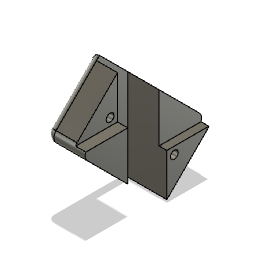
stepper mount v9 (Autodesk Fusion 360 design; units mm, degrees)
Autodesk Fusion 360 part; units mm, degrees
sketch "motor face" plane through (0, 0, 0) normal (0, 1, 0) x (1, 0, 0)
  circle A0 centre (0, 0) radius 14
  line L0 (0, 0) -> (37.537965, 0) construction
  circle A1 centre (17.5, 0) radius 2
  line L1 (17.5, 3.5) -> (13.555442, 3.5)
  line L2 (17.5, -3.5) -> (13.555442, -3.5)
  line L3 (0, 0) -> (0, 22.721675) construction
  circle A2 centre (0, 8) radius 4.5
  circle A3 centre (-17.5, 0) radius 2
  line L4 (-17.5, 3.5) -> (-13.555442, 3.5)
  line L5 (-17.5, -3.5) -> (-13.555442, -3.5)
  arc A4 (17.5, -3.5) -> (17.5, 3.5) centre (17.5, 0) ccw
  arc A5 (-17.5, 3.5) -> (-17.5, -3.5) centre (-17.5, 0) ccw
  line L6 (0, 0) -> (0, -28.412749) construction
  line L7 (0, -18) -> (8.8, -18)
  line L8 (8.8, -18) -> (8.8, -10.888526)
  line L9 (-8.8, -18) -> (-8.8, -10.888526)
  line L10 (0, -18) -> (-8.8, -18)
  circle A6 centre (0, 8) radius 2.46
  line L11 (-0.98, 10.256369) -> (-0.98, 5.743631)
  line L12 (0.98, 10.256369) -> (0.98, 5.743631)
  point P0 (0, 14)
  point P1 (0, 3.5)
  dimension "d1" = 28
  dimension "d2" = 4
  dimension "d3" = 17.5
  dimension "d4" = 7
  dimension "d5" = 9
  dimension "d6" = 10.5
  dimension "d7" = 8.8
  dimension "d8" = 32
  dimension "d11" = 4.92
  dimension "d12" = 0.98
  constraint coincident A0.centre L0.start
  constraint horizontal L0
  constraint coincident L0 A1.centre
  constraint concentric A1 A4
  constraint tangent L1 A4
  constraint horizontal L1
  constraint tangent L2 A4
  constraint parallel L1 L2
  constraint perpendicular L0 L3
  constraint coincident L3 A2.centre
  constraint coincident A0 P0
  constraint coincident L3 P0
  constraint coincident A2 P1
  constraint coincident L3 P1
  constraint symmetric A1 L3 A3
  constraint symmetric L3 A4 A5
  constraint symmetric L1.start L3 L4.start
  constraint symmetric L2.start L3 L5.start
  constraint perpendicular L0 L6
  constraint coincident L6 L7.start
  constraint perpendicular L6 L7
  constraint perpendicular L7 L8
  constraint symmetric L6 L7.start L10.start
  constraint symmetric L6 L7.end L9.start
  constraint concentric A2 A6
  constraint vertical L11
  measures "d1" diameter of A0
  measures "d2" diameter of A1
  measures "d3" distance of A0.centre A1.centre
  measures "d4" diameter of A4
  measures "d5" diameter of A2
  measures "d6" distance of P0 P1
  measures "d7" distance of L7.start L7.end
  measures "d8" distance of P0 L7
  measures "d11" diameter of A6
  measures "d12" distance of L3 L11
extrude "Extrude1" add sketch "motor face" along normal blind 19.3 contours A0 | A0 L7 L8 L9 L10 | A2 | A6 L12 | A6 L11 L12 | A6 L11 picked at (0.744544, -8.119418) picked at (4.18656, -16.495242) picked at (0, 11.811611) picked at (1.181596, 7.372833) picked at (-0.326667, 8.752123) picked at (-1.666309, 8.243546) makes body 1
extrude "Extrude2" add sketch "motor face" along normal blind 0.8 contours A0 L1 L2 A4 | A0 L4 L5 A5 picked at (15.851814, 2.910684) picked at (-15.851814, 2.910684) bodies 1
extrude "Extrude3" add sketch "motor face" against normal blind 1.34 contours A2 | A6 L12 | A6 L11 L12 | A6 L11 picked at (0, 11.811611) picked at (1.181596, 7.372833) picked at (-0.326667, 8.752123) picked at (-1.666309, 8.243546) bodies 1
extrude "Extrude4" add sketch "motor face" against normal blind 3.43 contours A6 L12 | A6 L11 L12 | A6 L11 picked at (1.181596, 7.372833) picked at (-0.326667, 8.752123) picked at (-1.666309, 8.243546) bodies 1
extrude "Extrude5" add sketch "motor face" against normal blind 9.43 contours A6 L11 L12 picked at (-0.326667, 8.752123) bodies 1
sketch "motor clamp face" plane through (0, 0, 0) normal (0, 1, 0) x (1, 0, 0)
  circle A0 centre (17.5, 0) radius 2
  line L0 (17.5, 3.5) -> (13.555442, 3.5)
  arc A1 (17.5, -3.5) -> (17.5, 3.5) centre (17.5, 0) ccw
  line L1 (17.5, -3.5) -> (13.555442, -3.5)
  arc A2 (13.555442, 3.5) -> (-13.555442, 3.5) centre (0, 0) ccw
  arc A3 (-13.555442, -3.5) -> (-8.8, -10.888526) centre (0, 0) ccw
  arc A4 (8.8, -10.888526) -> (13.555442, -3.5) centre (0, 0) ccw
  circle A5 centre (-17.5, 0) radius 2
  line L2 (-17.5, -3.5) -> (-13.555442, -3.5)
  arc A6 (-17.5, 3.5) -> (-17.5, -3.5) centre (-17.5, 0) ccw
  line L3 (-17.5, 3.5) -> (-13.555442, 3.5)
  line L4 (8.8, -18) -> (-8.8, -18)
  line L5 (-8.8, -18) -> (-8.8, -10.888526)
  line L6 (8.8, -18) -> (8.8, -10.888526)
  circle A7 centre (0, 0) radius 22
  line L7 (-22, 10) -> (22, 10)
  line L8 (22, 10) -> (22, -10)
  line L9 (22, -10) -> (-22, -10)
  line L10 (-22, -10) -> (-22, 10)
  line L11 (-22, 10) -> (22, -10) construction
  line L12 (22, 10) -> (-22, -10) construction
  circle A8 centre (17.5, 0) radius 1.25
  circle A9 centre (-17.5, 0) radius 1.25
  dimension "d21" = 20
  dimension "d25" = 44
  dimension "d27" = 2.5
  dimension "d28" = 2.5
  constraint concentric A2 A7
  constraint horizontal L7
  constraint perpendicular L7 L8
  constraint parallel L7 L9
  constraint parallel L8 L10
  constraint coincident L11 A2.centre
  constraint coincident L12 A2.centre
  constraint coincident A2.centre A3.centre
  constraint tangent A7 L10
  constraint concentric A0 A8
  constraint concentric A5 A9
  measures "d21" distance of L7.end L8.end
  measures "d25" distance of L7.start L7.end
  measures "d27" diameter of A8
  measures "d28" diameter of A9
extrude "Extrude6" add sketch "motor clamp face" along normal blind 40 separate body contours A0 | L0 A1 L1 A2 A3 A4 L2 A6 L3 L7 L9 | L0 A1 L1 A2 A4 A7 L7 L9 | A2 A3 L2 A6 L3 A7 L7 L9 | A5 | A8 | A9 picked at (19.2379, -0.161462) picked at (-3.265986, 3.333333) picked at (16.684362, -6.267352) picked at (-16.684362, -6.267352) picked at (-15.7621, -0.161462) picked at (17.867018, -0.068883) picked at (-17.132982, -0.068883) makes body 2
combine "Combine1" operation cut target body 2 tool bodies 1 keep tools
move_face "OffsetFaces1" offset -0.3 9 faces at (12.790197, 12.866667, 5.693053) (-3.265986, 19.3, -3.333333) (16.185147, 0.266667, 3.5) (19.325023, 0.266667, -2.986518) (16.185147, 0.266667, -3.5) (-12.790197, 12.866667, -5.693053) (-16.185147, 0.266667, -3.5) (-19.325023, 0.266667, 2.986518) (-16.185147, 0.266667, 3.5) on bodies 2
move_face "OffsetFaces2" offset -0.8 2 faces at (-16.978792, 0, -0.179043) (18.166667, 0, 0.578512) on bodies 2
extrude "Extrude7" cut sketch "motor clamp face" along normal blind 20 contours A8 | A9 picked at (17.867018, -0.068883) picked at (-17.132982, -0.068883) bodies 2
sketch "bar clamp face" plane through (0, 40, 0) normal (0, 1, 0) x (-1, 0, 0)
  arc A0 (19.595918, -10) -> (19.595918, 10) centre (0, 0) ccw
  line L0 (19.595918, 10) -> (-19.595918, 10)
  arc A1 (-19.595918, 10) -> (-19.595918, -10) centre (0, 0) ccw
  line L1 (-19.595918, -10) -> (19.595918, -10)
  line L2 (-6.35, 6.35) -> (6.35, 6.35)
  line L3 (6.35, 6.35) -> (6.35, -6.35)
  line L4 (6.35, -6.35) -> (-6.35, -6.35)
  line L5 (-6.35, -6.35) -> (-6.35, 6.35)
  line L6 (-6.35, 6.35) -> (6.35, -6.35) construction
  line L7 (6.35, 6.35) -> (-6.35, -6.35) construction
  line L8 (-22, 0.5) -> (22, 0.5)
  line L9 (22, 0.5) -> (22, -0.5)
  line L10 (22, -0.5) -> (-22, -0.5)
  line L11 (-22, -0.5) -> (-22, 0.5)
  line L12 (-22, 0.5) -> (22, -0.5) construction
  line L13 (22, 0.5) -> (-22, -0.5) construction
  dimension "d33" = 12.7
  dimension "d34" = 12.7
  dimension "d35" = 1
  constraint horizontal L2
  constraint perpendicular L2 L3
  constraint parallel L2 L4
  constraint parallel L3 L5
  constraint coincident L6 A0.centre
  constraint coincident L7 A0.centre
  constraint coincident A0.centre A1.centre
  constraint horizontal L8
  constraint perpendicular L8 L9
  constraint parallel L8 L10
  constraint parallel L9 L11
  constraint coincident L12 A0.centre
  constraint coincident L13 A0.centre
  constraint tangent A1 L11
  measures "d33" distance of L3.end L4.end
  measures "d34" distance of L2.end L3.end
  measures "d35" distance of L8.end L9.end
extrude "Extrude8" cut sketch "bar clamp face" against normal up to surface (20.4 mm away) contours A0 L3 L8 L10 | L3 L5 L8 L10 | L3 L4 L5 L10 | A1 L5 L8 L10 | L2 L3 L5 L8 picked at (11.566667, 0) picked at (2.116667, -0.166667) picked at (-2.116667, -2.45) picked at (-11.566667, 0) picked at (2.116667, 2.45) bodies 2
sketch "bar clamp bolts" plane through (0, 0, -10) normal (0, 0, -1) x (-1, 0, 0)
  line L0 (-10.222035, 0) -> (-10.222035, 19.6)
  line L1 (-10.222035, 19.6) -> (10.222035, 19.6)
  line L2 (10.222035, 19.6) -> (10.222035, 0)
  line L3 (10.222035, 0) -> (19.595918, 0)
  line L4 (19.595918, 0) -> (19.595918, 40)
  line L5 (19.595918, 40) -> (-19.595918, 40)
  line L6 (-19.595918, 40) -> (-19.595918, 0)
  line L7 (-19.595918, 0) -> (-10.222035, 0)
  line L8 (-6.35, 19.6) -> (6.35, 19.6)
  line L9 (6.35, 19.6) -> (6.35, 40)
  line L10 (6.35, 40) -> (-6.35, 40)
  line L11 (-6.35, 40) -> (-6.35, 19.6)
  circle A0 centre (-11.493103, 31) radius 1.6
  circle A1 centre (-11.493103, 31) radius 3
  line L12 (-11.493103, 31) -> (-11.493103, 34) construction
  line L13 (-11.493103, 31) -> (-8.35, 31) construction
  line L14 (0, 1.75) -> (0, 22.5)
  circle A2 centre (11.493103, 31) radius 1.6
  circle A3 centre (11.493103, 31) radius 3
  point P0 (-8.493103, 31)
  point P1 (-11.493103, 34)
  dimension "d38" = 3.2
  dimension "d39" = 6
  dimension "d40" = 6
  dimension "d41" = 2
  constraint concentric A0 A1
  constraint vertical L12
  constraint perpendicular L12 L13
  constraint symmetric A0 L14 A2
  constraint symmetric A1 L14 A3
  measures "d38" diameter of A0
  measures "d39" diameter of A1
  measures "d41" distance of L11 L13.end
extrude "Extrude9" cut sketch "bar clamp bolts" against normal up to surface (20 mm away) contours A0 | A2 picked at (-11.453247, 30.608082) picked at (11.532959, 30.608082) bodies 2
extrude "Extrude10" cut sketch "bar clamp bolts" against normal blind 1 contours A1 | A3 picked at (-8.976895, 30.771469) picked at (14.00931, 30.771469) bodies 2
sketch "bar clamp nuts" plane through (0, 0, 10) normal (0, 0, 1) x (1, 0, 0)
  circle A0 centre (11.493103, 31) radius 1.6
  circle A1 centre (-11.493103, 31) radius 1.6
  line L0 (10.222035, 19.6) -> (10.222035, 0)
  line L1 (10.222035, 0) -> (19.595918, 0)
  line L2 (19.595918, 0) -> (19.595918, 40)
  line L3 (19.595918, 40) -> (-19.595918, 40)
  line L4 (-19.595918, 40) -> (-19.595918, 0)
  line L5 (-19.595918, 0) -> (-10.222035, 0)
  line L6 (-10.222035, 0) -> (-10.222035, 19.6)
  line L7 (-10.222035, 19.6) -> (10.222035, 19.6)
  circle A2 centre (-11.493103, 31) radius 3
  circle A3 centre (11.493103, 31) radius 3
  dimension "d46" = 6
  dimension "d47" = 6
  constraint concentric A1 A2
  constraint concentric A0 A3
  measures "d46" diameter of A2
  measures "d47" diameter of A3
extrude "Extrude11" cut sketch "bar clamp nuts" against normal blind 1 contours A2 | A3 picked at (-8.970939, 30.850958) picked at (14.00931, 30.771469) bodies 2
chamfer "Chamfer1" distance 1 angle 45 6 edges at (0, 40, -6.35) (-6.35, 40, -3.425) (6.35, 40, -3.425) (6.35, 40, 3.425) (0, 40, 6.35) (-6.35, 40, 3.425) on bodies 2
fillet "Fillet1" radius 4 10 edges at (19.595918, 20, -10) (-19.595918, 20, -10) (0, 40, -10) (19.595918, 20, 10) (21.330715, 40, 5.385219) (21.330715, 40, -5.385219) (0, 40, 10) (-19.595918, 20, 10) (-21.330715, 40, -5.385219) (-21.330715, 40, 5.385219) on bodies 2
extrude "Extrude12" add sketch "bar clamp face" along normal blind 100 separate body contours L3 L5 L8 L10 | L3 L4 L5 L10 | L2 L3 L5 L8 picked at (2.116667, -0.166667) picked at (-2.116667, -2.45) picked at (2.116667, 2.45) makes body 3
sketch "v bar" plane through (0, 0, 6.35) normal (0, 0, 1) x (1, 0, 0)
  line L0 (-6.35, 40) -> (6.35, 40)
  line L1 (6.35, 40) -> (6.35, 140)
  line L2 (6.35, 140) -> (-6.35, 140)
  line L3 (-6.35, 140) -> (-6.35, 40)
  line L4 (19.05, 90) -> (6.35, 90)
  line L5 (6.35, 90) -> (6.35, 102.7)
  line L6 (6.35, 102.7) -> (19.05, 102.7)
  line L7 (19.05, 102.7) -> (19.05, 90)
  line L8 (19.05, 90) -> (6.35, 102.7) construction
  line L9 (6.35, 90) -> (19.05, 102.7) construction
  line L10 (6.35, 40) -> (-6.35, 40)
  point P0 (12.7, 96.35)
  dimension "d55" = 12.7
  dimension "d56" = 12.7
  dimension "d57" = 50
  constraint horizontal L4
  constraint perpendicular L4 L5
  constraint parallel L4 L6
  constraint parallel L5 L7
  constraint coincident L8 P0
  constraint coincident L9 P0
  constraint collinear L1 L5
  measures "d55" distance of L5.end L6.end
  measures "d56" distance of L4.end L5.end
  measures "d57" distance of L4 L10
extrude "Extrude13" add sketch "v bar" along normal mid plane 100 separate body contours L1 L4 L5 L6 L7 picked at (10.583333, 98.466667) makes body 4
sketch "A clamp bolts" plane through (6.35, 0, 0) normal (1, 0, 0) x (0, 0, -1)
  line L0 (-6.35, 40) -> (6.35, 40)
  line L1 (6.35, 40) -> (6.35, 140)
  line L2 (6.35, 140) -> (-6.35, 140)
  line L3 (-6.35, 140) -> (-6.35, 40)
  line L4 (43.65, 102.7) -> (-56.35, 102.7)
  line L5 (-56.35, 102.7) -> (-56.35, 90)
  line L6 (-56.35, 90) -> (43.65, 90)
  line L7 (43.65, 90) -> (43.65, 102.7)
  circle A0 centre (11.35, 107.7) radius 3 construction
  circle A1 centre (11.35, 107.7) radius 1.6
  line L8 (6.35, 112.7) -> (16.35, 112.7)
  line L9 (16.35, 112.7) -> (16.35, 102.7)
  line L10 (0, 40) -> (0, 140) construction
  line L11 (-56.35, 96.35) -> (43.65, 96.35) construction
  line L12 (-6.35, 112.7) -> (-16.35, 112.7)
  line L13 (-16.35, 112.7) -> (-16.35, 102.7)
  circle A2 centre (-11.35, 107.7) radius 1.6
  circle A3 centre (-11.35, 85) radius 1.6
  line L14 (-6.35, 80) -> (-16.35, 80)
  line L15 (-16.35, 80) -> (-16.35, 90)
  line L16 (6.35, 80) -> (16.35, 80)
  circle A4 centre (11.35, 85) radius 1.6
  line L17 (16.35, 80) -> (16.35, 90)
  line L18 (6.35, 112.7) -> (-6.35, 112.7)
  line L19 (16.35, 102.7) -> (16.35, 90)
  line L20 (6.35, 80) -> (-6.35, 80)
  line L21 (-16.35, 102.7) -> (-16.35, 90)
  circle A5 centre (-11.35, 107.7) radius 3
  circle A6 centre (11.35, 85) radius 3
  line L22 (-14.1, 83.412287) -> (-11.35, 81.824574)
  line L23 (-11.35, 81.824574) -> (-8.6, 83.412287)
  line L24 (-8.6, 83.412287) -> (-8.6, 86.587713)
  line L25 (-8.6, 86.587713) -> (-11.35, 88.175426)
  line L26 (-11.35, 88.175426) -> (-14.1, 86.587713)
  line L27 (-14.1, 86.587713) -> (-14.1, 83.412287)
  line L28 (8.6, 106.112287) -> (11.35, 104.524574)
  line L29 (11.35, 104.524574) -> (14.1, 106.112287)
  line L30 (14.1, 106.112287) -> (14.1, 109.287713)
  line L31 (14.1, 109.287713) -> (11.35, 110.875426)
  line L32 (11.35, 110.875426) -> (8.6, 109.287713)
  line L33 (8.6, 109.287713) -> (8.6, 106.112287)
  point P0 (8.35, 107.7)
  point P1 (11.35, 104.7)
  point P2 (11.35, 110.7)
  point P3 (14.35, 107.7)
  point P4 (-11.35, 85)
  point P5 (11.35, 107.7)
  dimension "d60" = 6
  dimension "d61" = 3.2
  dimension "d62" = 2
  dimension "d63" = 2
  dimension "d64" = 2
  dimension "d65" = 2
  dimension "d71" = 6
  dimension "d72" = 6
  dimension "d73" = 2.75
  dimension "d74" = 2.75
  constraint concentric A0 A1
  constraint coincident A0 P0
  constraint coincident A0 P1
  constraint coincident L1 L8.start
  constraint perpendicular L1 L8
  constraint coincident L4 L9.end
  constraint perpendicular L4 L9
  constraint coincident A0 P2
  constraint coincident A0 P3
  constraint midpoint L0 L10.start
  constraint midpoint L2 L10.end
  constraint midpoint L5 L11.start
  constraint midpoint L7 L11.end
  constraint symmetric A1 L10 A2
  constraint symmetric L8.start L10 L12.start
  constraint symmetric L8.end L10 L12.end
  constraint symmetric L9.end L10 L13.end
  constraint symmetric A1 L11 A4
  constraint symmetric L8.start L11 L16.start
  constraint symmetric L8.end L11 L16.end
  constraint symmetric L9.end L11 L17.end
  constraint symmetric L11 L12.start L14.start
  constraint symmetric L11 L12.end L14.end
  constraint symmetric L11 L13.end L15.end
  constraint symmetric L11 A2 A3
  constraint concentric A2 A5
  constraint concentric A4 A6
  constraint coincident P4 A3.centre
  constraint coincident P5 A0.centre
  measures "d60" diameter of A0
  measures "d61" diameter of A1
  measures "d62" distance of L1 P0
  measures "d63" distance of L4 P1
  measures "d64" distance of L9 P3
  measures "d65" distance of L8 P2
  measures "d71" diameter of A5
  measures "d72" diameter of A6
  measures "d73" distance of P4 L27
  measures "d74" distance of P5 L33
extrude "Extrude14" add sketch "A clamp bolts" along normal blind 15.7 separate body contours L3 L6 L14 L15 | L1 L3 L6 L20 | L1 L6 L16 L17 | L3 L4 L6 L21 | L1 L3 L4 L6 | L1 L4 L6 L19 | L3 L4 L12 L13 | L1 L3 L4 L18 | L1 L4 L8 L9 | A5 | A6 | L22 L23 L24 L25 L26 L27 | L28 L29 L30 L31 L32 L33 picked at (-15.6, 84.470762) picked at (2.116667, 83.333333) picked at (11.27527, 80.669463) picked at (-13.016667, 94.233333) picked at (-2.116667, 98.466667) picked at (13.016667, 98.466667) picked at (-11.42473, 103.369463) picked at (-2.116667, 109.366667) picked at (7.1, 107.170762) picked at (-9.012942, 106.739956) picked at (13.687058, 84.039956) picked at (-10.166667, 82.950407) picked at (12.533333, 109.749593) makes body 5
combine "Combine2" operation cut target body 5 tool bodies 4 keep tools
move_face "OffsetFaces3" offset -0.3 2 faces at (6.35, 81.170201, 3.588485) (6.35, 103.870201, 3.588485) on bodies 5
fillet "Fillet2" radius 3 8 edges at (14.35, 112.7, 16.35) (22.05, 96.35, 16.35) (22.05, 112.7, 0) (22.05, 80, 0) (14.35, 80, 16.35) (14.35, 80, -16.35) (22.05, 96.35, -16.35) (14.35, 112.7, -16.35) on bodies 5
extrude "Extrude15" cut sketch "A clamp bolts" along normal blind 20 from surface at 11 contours A5 | A6 | L22 L23 L24 L25 L26 L27 | L28 L29 L30 L31 L32 L33 picked at (-9.012942, 106.739956) picked at (13.687058, 84.039956) picked at (-10.166667, 82.950407) picked at (12.533333, 109.749593) bodies 5
mirror "Mirror1" about plane through (6.35, 90, 6.35) normal (-1, 0, 0) of bodies 5 makes body 6
sketch "B clamp" plane through (6.35, 0, 0) normal (-1, 0, 0) x (0, 0, 1)
  line L0 (-43.65, 90) -> (56.35, 90)
  line L1 (56.35, 90) -> (56.35, 102.7)
  line L2 (56.35, 102.7) -> (-43.65, 102.7)
  line L3 (-43.65, 102.7) -> (-43.65, 90)
  line L4 (-43.65, 102.7) -> (-43.65, 90)
  line L5 (56.35, 102.7) -> (-43.65, 102.7)
  line L6 (56.35, 90) -> (56.35, 102.7)
  line L7 (-43.65, 90) -> (56.35, 90)
  line L8 (-6.35, 40) -> (6.35, 40)
  line L9 (-6.35, 40) -> (-6.35, 140)
  line L10 (6.35, 140) -> (-6.35, 140)
  line L11 (6.35, 40) -> (6.35, 140)
  circle A0 centre (9.35, 105.7) radius 3
  line L12 (-43.65, 96.35) -> (56.35, 96.35) construction
  line L13 (0, 140) -> (0, 40) construction
  line L14 (0, 96.35) -> (49.007667, 47.342333) construction
  line L15 (9.885534, 86.464466) -> (35.405807, 111.984739)
  line L16 (0, 96.35) -> (34.507271, 130.857271) construction
  line L17 (15.006854, 111.356854) -> (24.892388, 101.47132)
  circle A1 centre (9.35, 105.7) radius 1.6
  circle A2 centre (9.35, 105.7) radius 1.1
  line L18 (-9.885534, 106.235534) -> (15.634739, 131.755807)
  line L19 (15.006854, 111.356854) -> (5.12132, 121.242388)
  line L20 (9.885534, 86.464466) -> (-15.634739, 60.944193)
  line L21 (-15.006854, 81.343146) -> (-5.12132, 71.457612)
  line L22 (-9.885534, 106.235534) -> (-35.405807, 80.715261)
  circle A3 centre (-9.35, 87) radius 3
  circle A4 centre (-9.35, 87) radius 1.6
  circle A5 centre (-9.35, 87) radius 1.1
  line L23 (-15.006854, 81.343146) -> (-24.892388, 91.22868)
  line L24 (6.35, 103.967949) -> (9.35, 102.235898)
  line L25 (9.35, 102.235898) -> (12.35, 103.967949)
  line L26 (12.35, 103.967949) -> (12.35, 107.432051)
  line L27 (12.35, 107.432051) -> (9.35, 109.164102)
  line L28 (9.35, 109.164102) -> (6.35, 107.432051)
  line L29 (6.35, 107.432051) -> (6.35, 103.967949)
  point P0 (6.35, 90)
  point P1 (9.885534, 86.464466)
  point P2 (9.35, 105.7)
  dimension "d80" = 6
  dimension "d81" = 135
  dimension "d82" = 5
  dimension "d83" = 8
  dimension "d84" = 3.2
  dimension "d85" = 2.2
  dimension "d137" = 3
  constraint tangent L11 A0
  constraint tangent L2 A0
  constraint midpoint L4 L12.start
  constraint midpoint L6 L12.end
  constraint midpoint L10 L13.start
  constraint midpoint L8 L13.end
  constraint coincident L12 L14.start
  constraint coincident L13 L14.start
  constraint perpendicular L14 L15
  constraint midpoint L7 P0
  constraint perpendicular L14 L16
  constraint perpendicular L15 L17
  constraint concentric A0 A1
  constraint concentric A1 A2
  constraint symmetric A0 L14 A3
  constraint symmetric L14 A1 A4
  constraint symmetric L14 A2 A5
  constraint coincident P2 A0.centre
  measures "d80" diameter of A0
  measures "d81" angle of L13 L14
  measures "d84" diameter of A1
  measures "d85" diameter of A2
  measures "d137" distance of P2 L29
extrude "Extrude16" add sketch "B clamp" along normal blind 15.7 separate body contours L0 L2 L5 L7 L9 L22 L23 | L0 L7 L9 L21 A3 L23 | L2 L5 L9 L18 L22 | L0 L7 L9 A3 | A3 | L2 L5 L9 L11 L18 L19 L29 | L0 L2 L5 L7 L9 L11 | L0 L7 L9 L11 L20 L21 | L2 L5 L11 L24 | L0 L2 L5 L7 L11 L15 L17 L24 L25 | L0 L7 L11 L15 L20 | L2 L5 A0 L24 | L2 L5 L24 L25 | L11 A0 L24 L29 | L2 L5 A0 L25 | A0 | L11 A0 L28 L29 | L2 L5 L11 L17 L19 L25 L26 L27 L28 | A0 L25 L26 | A0 L27 L28 | A0 L26 L27 picked at (-15.478259, 94.233333) picked at (-10.284686, 79.34435) picked at (-7.528511, 106.235534) picked at (-6.93939, 89.41061) picked at (-9.536587, 89.521019) picked at (2.116667, 112.405609) picked at (-2.116667, 98.466667) picked at (-2.116667, 80.871741) picked at (6.85, 103.256624) picked at (15.746208, 98.466667) picked at (9.885534, 88.821489) picked at (8.692706, 102.742629) picked at (9.617949, 102.545299) picked at (6.622792, 104.125446) picked at (10.007294, 102.742629) picked at (8.217992, 107.958779) picked at (6.622792, 107.274554) picked at (17.006854, 106.585618) picked at (12.077208, 104.125446) picked at (9.35, 108.849108) picked at (12.077208, 107.274554) makes body 7
combine "Combine3" operation cut target body 7 tool bodies 3 keep tools
extrude "Extrude19" add sketch "B clamp" against normal blind 3.175 contours L0 L7 L9 L21 A3 L23 | L0 L7 L9 A3 | A3 | A4 | A5 picked at (-10.284686, 79.34435) picked at (-6.93939, 89.41061) picked at (-9.536587, 89.521019) picked at (-8.125868, 86.261607) picked at (-9.216042, 86.65868) bodies 7
extrude "Extrude20" cut sketch "B clamp" along normal blind 4.175 contours L2 L5 L11 L24 | L2 L5 A0 L24 | L11 A0 L24 L29 | L2 L5 A0 L25 | A0 | L11 A0 L28 L29 | L2 L5 L11 L17 L19 L25 L26 L27 L28 | A0 L25 L26 | A0 L27 L28 | A0 L26 L27 | A1 | A2 picked at (6.85, 103.256624) picked at (8.692706, 102.742629) picked at (6.622792, 104.125446) picked at (10.007294, 102.742629) picked at (8.217992, 107.958779) picked at (6.622792, 107.274554) picked at (17.006854, 106.585618) picked at (12.077208, 104.125446) picked at (9.35, 108.849108) picked at (12.077208, 107.274554) picked at (10.574132, 104.961607) picked at (9.483958, 105.35868) bodies 7
extrude "Extrude21" cut sketch "B clamp" against normal blind 2 from surface at 15.7 contours A3 | L2 L5 A0 L24 | L2 L5 L24 L25 | L11 A0 L24 L29 | L2 L5 A0 L25 | A0 | L11 A0 L28 L29 | A0 L25 L26 | A0 L27 L28 | A0 L26 L27 | A4 | A5 picked at (-9.536587, 89.521019) picked at (8.692706, 102.742629) picked at (9.617949, 102.545299) picked at (6.622792, 104.125446) picked at (10.007294, 102.742629) picked at (8.217992, 107.958779) picked at (6.622792, 107.274554) picked at (12.077208, 104.125446) picked at (9.35, 108.849108) picked at (12.077208, 107.274554) picked at (-8.125868, 86.261607) picked at (-9.216042, 86.65868) bodies 7
extrude "Extrude22" cut sketch "B clamp" along normal mid plane 100 contours A4 | A5 picked at (-8.125868, 86.261607) picked at (-9.216042, 86.65868) bodies 7
fillet "Fillet3" radius 3 6 edges at (-9.35, 106.235534, -9.885534) (-9.35, 86.464466, 9.885534) (-9.35, 111.356854, 15.006854) (-9.35, 81.343146, -15.006854) (-1.5, 101.47132, 24.892388) (-1.5, 91.22868, -24.892388) on bodies 7
sketch "base clamp layout" plane through (0, 0, 56.35) normal (0, 0, 1) x (1, 0, 0)
  line L0 (19.05, 102.7) -> (6.35, 102.7)
  line L1 (6.35, 102.7) -> (6.35, 90)
  line L2 (6.35, 90) -> (19.05, 90)
  line L3 (19.05, 90) -> (19.05, 102.7)
  line L4 (6.35, 102.7) -> (19.05, 102.7)
  line L5 (19.05, 102.7) -> (19.05, 90)
  line L6 (19.05, 90) -> (6.35, 90)
  line L7 (6.35, 90) -> (6.35, 102.7)
  line L8 (19.05, 102.7) -> (-29.385671, 54.264329) construction
  line L9 (19.05, 102.7) -> (87.548383, 102.7) construction
  line L10 (19.05, 90) -> (6.35, 102.7) construction
  circle A0 centre (12.7, 96.35) radius 14.980256
  line L11 (4.935786, 88.585786) -> (-2.269838, 95.791411) construction
  line L12 (1.545866, 86.350331) -> (22.699669, 107.504134)
  line L13 (12.7, 96.35) -> (-15.230923, 96.35) construction
  circle A1 centre (-5.280256, 96.35) radius 3 construction
  circle A2 centre (-5.280256, 96.35) radius 1.6
  circle A3 centre (12.7, 114.330256) radius 1.6
  circle A4 centre (12.7, 96.35) radius 20.980256
  line L14 (1.545866, 86.350331) -> (-5.922609, 78.881856)
  line L15 (22.699669, 107.504134) -> (30.5569, 115.361365)
  circle A5 centre (12.7, 78.369744) radius 1.6
  circle A6 centre (30.680256, 96.35) radius 1.6
  point P0 (2.107359, 85.757359)
  point P1 (4.935786, 88.585786)
  dimension "d105" = 135
  dimension "d106" = 2
  dimension "d107" = 4
  dimension "d120" = 6
  dimension "d121" = 3.2
  constraint horizontal L9
  constraint coincident L0.start L3.end
  constraint coincident L2.end L3.start
  constraint coincident L0.end L1.start
  constraint midpoint L10 A0.centre
  constraint perpendicular L8 L11
  constraint perpendicular L10 L12
  constraint coincident A0.centre L13.start
  constraint horizontal L13
  constraint tangent A0 A1
  constraint concentric A1 A2
  constraint symmetric L10 A2 A3
  constraint concentric A0 A4
  constraint tangent A1 A4
  constraint parallel L12 L14
  constraint parallel L12 L15
  constraint symmetric L8 A2 A5
  constraint symmetric L8 A3 A6
  measures "d105" angle of L8 L9
  measures "d120" diameter of A1
  measures "d121" diameter of A2
extrude "Extrude23" add sketch "base clamp layout" against normal blind 12 separate body contours L0 L1 L4 L7 A0 L12 picked at (3.519062, 97.409687) makes body 8
sketch "base clamp bolts" plane through (-42.402233, 42.402233, 0) normal (0.707107, -0.707107, 0) x (0, 0, -1)
  line L0 (-56.35, 68.946068) -> (-56.35, 62.151997)
  line L1 (-56.35, 62.151997) -> (-44.35, 62.151997)
  line L2 (-44.35, 62.151997) -> (-44.35, 68.946068)
  line L3 (-44.35, 68.946068) -> (-56.35, 68.946068)
  line L4 (-56.35, 66.129738) -> (-44.35, 66.129738) construction
  circle A0 centre (-50.35, 66.129738) radius 1.6
  circle A1 centre (-50.35, 66.129738) radius 3
  circle A2 centre (-50.35, 66.129738) radius 1.1
  line L5 (-56.35, 77.109994) -> (-43.033126, 77.109994) construction
  circle A3 centre (-50.35, 88.090251) radius 1.1
  point P0 (-56.35, 66.129738)
  point P1 (-56.35, 66.129738)
  point P2 (-50.35, 66.129738)
  point P3 (-56.35, 77.109994)
  dimension "d110" = 3.2
  dimension "d111" = 6
  dimension "d112" = 2.2
  constraint perpendicular L2 L4
  constraint concentric A0 A1
  constraint concentric A1 A2
  constraint horizontal L5
  constraint symmetric A2 L5 A3
  measures "d110" diameter of A0
  measures "d111" diameter of A1
  measures "d112" diameter of A2
extrude "Extrude24" cut sketch "base clamp bolts" against normal blind 30 contours A3 picked at (-50.066585, 88.376922) bodies 8
extrude "Extrude25" cut sketch "base clamp bolts" against normal blind 30 contours A0 | A2 picked at (-49.397898, 67.196145) picked at (-50.633415, 65.843067) bodies 8
extrude "Extrude27" add sketch "base clamp layout" against normal blind 3 contours A0 A4 L14 L15 picked at (-4.690027, 92.228281) bodies 8
fillet "Fillet4" radius 3 1 edges at (2.107359, 106.942641, 53.35) on bodies 8
extrude "Extrude26" cut sketch "base clamp bolts" against normal blind 20 from surface at -5 contours L3 A1 | L3 A1 picked at (-50.559477, 68.985105) picked at (-50.389856, 68.539134) bodies 8
sketch "Base bolt counterbores" plane through (0, 0, 53.35) normal (0, 0, -1) x (-1, 0, 0)
  arc A0 (2.70128, 82.103185) -> (-26.946815, 111.75128) centre (-12.7, 96.35) ccw
  line L0 (-26.946815, 111.75128) -> (-24.823618, 109.628083)
  arc A1 (-14.298415, 114.259067) -> (-24.823618, 109.628083) centre (-12.7, 96.35) ccw
  arc A2 (-11.101585, 114.259067) -> (-14.298415, 114.259067) centre (-12.7, 114.330256) ccw
  arc A3 (5.132073, 98.653646) -> (-11.101585, 114.259067) centre (-12.7, 96.35) ccw
  arc A4 (5.209067, 97.948415) -> (5.132073, 98.653646) centre (-12.7, 96.35) ccw
  arc A5 (5.209067, 94.751585) -> (5.209067, 97.948415) centre (5.280256, 96.35) ccw
  arc A6 (0.578083, 84.226382) -> (5.209067, 94.751585) centre (-12.7, 96.35) ccw
  line L1 (0.578083, 84.226382) -> (2.70128, 82.103185)
  circle A7 centre (-12.7, 114.330256) radius 3
  circle A8 centre (5.280256, 96.35) radius 3
  dimension "d126" = 6
  dimension "d127" = 6
  constraint concentric A2 A7
  constraint concentric A5 A8
  measures "d126" diameter of A7
  measures "d127" diameter of A8
extrude "Extrude28" cut sketch "Base bolt counterbores" along normal blind 4 contours A3 A4 A5 A6 A8 | A1 A2 A3 A7 | A3 A4 A5 A6 A8 | A1 A2 A3 A7 picked at (5.562991, 98.538085) picked at (-10.535771, 114.70391) picked at (4.232797, 96.35) picked at (-12.7, 113.282797) bodies 8
fillet "Fillet5" radius 1 2 edges at (-2.135281, 111.185281, 53.35) (2.107359, 106.942641, 44.35) on bodies 8
sketch "baseplate" plane through (0, 0, 0) normal (0, 0, 1) x (1, 0, 0)
  circle A0 centre (12.7, 78.369744) radius 1.6
  circle A1 centre (30.680256, 96.35) radius 1.6
  circle A2 centre (12.7, 114.330256) radius 1.6
  circle A3 centre (-5.280256, 96.35) radius 1.6
  line L0 (-40, -20.669744) -> (40, -20.669744)
  line L1 (50, -10.669744) -> (50, 119.330256)
  line L2 (40, 129.330256) -> (-40, 129.330256)
  line L3 (-50, 119.330256) -> (-50, -10.669744)
  line L4 (0, 1.75) -> (0, 22.5)
  arc A4 (-50, -10.669744) -> (-40, -20.669744) centre (-40, -10.669744) ccw
  arc A5 (40, -20.669744) -> (50, -10.669744) centre (40, -10.669744) ccw
  arc A6 (50, 119.330256) -> (40, 129.330256) centre (40, 119.330256) ccw
  arc A7 (-40, 129.330256) -> (-50, 119.330256) centre (-40, 119.330256) ccw
  point P0 (12.7, 114.330256)
  point P1 (-50, -20.669744)
  point P2 (50, -20.669744)
  point P3 (50, 129.330256)
  dimension "d132" = 100
  dimension "d133" = 150
  dimension "d134" = 50
  dimension "d135" = 15
  dimension "d136" = 10
  constraint horizontal L0
  constraint vertical L1
  constraint horizontal L2
  constraint vertical L3
  constraint tangent L0 A4
  constraint tangent L3 A4
  constraint tangent L0 A5
  constraint tangent L1 A5
  constraint equal A4 A5
  constraint tangent L1 A6
  constraint tangent L2 A6
  constraint equal A4 A6
  constraint tangent L2 A7
  constraint tangent L3 A7
  constraint equal A4 A7
  measures "d134" distance of L1 L4
  measures "d136" radius of A4
hidden bodies 1 2 3 4 5 6 8
equation "d3 = ( ( 39 - 4 ) / 2 ) * 1 mm"
equation "d7 = ( 17.6 / 2 ) * 1 mm"
equation "d12 = ( ( 4.92 - 2.96 ) / 2 ) * 1 mm"
equation "motorClearance = 0.3 mm"
equation "d26 = -motorClearance"
equation "tubeWidth = 12.7 mm"
equation "d33 = tubeWidth"
equation "d34 = tubeWidth"
equation "d55 = tubeWidth"
equation "d56 = tubeWidth"
equation "d66 = tubeWidth + 3 mm"
equation "d73 = ( 5.5 / 2 ) * 1 mm"
equation "d74 = ( 5.5 / 2 ) * 1 mm"
equation "d86 = tubeWidth + 3 mm"
equation "d94 = -tubeWidth / 4"
equation "d96 = tubeWidth / 4 + 1 mm"
named bodies: "28BYJ-48", "stepper mount", "h bar", "v bar", "A clamp1", "A clamp2", "B clamp", "base clamp"
